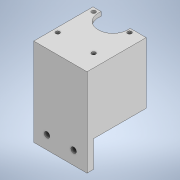
# Autodesk Inventor part: サーボモータ固定用
Saved by Autodesk Inventor 2022 (Build 260153000, 153)
## iProperties
Created: 2022-11-22
Part Number: サーボモータ固定用
Material: 一般
Document SubType Name: Modeling
Designer: tdn82
Density: 1 g/cm^3
Appearance: 既定
Author: tdn82
Autodesk Inventor part; units mm, degrees
ref_plane "YZ Plane" through (0, 0, 0) normal (1, 0, 0) x (0, 1, 0)
ref_plane "XZ Plane" through (0, 0, 0) normal (0, 1, 0) x (-1, 0, 0)
ref_plane "XY Plane" through (0, 0, 0) normal (0, 0, 1) x (1, 0, 0)
sketch "スケッチ1" plane through (0, 0, 0) normal (0, 1, 0) x (-1, 0, 0)
  line L0 (0, 0) -> (-34, 0)
  line L1 (-34, 0) -> (-34, -44.5)
  line L2 (-34, -44.5) -> (0, -44.5)
  line L3 (0, -44.5) -> (0, 0)
  dimension "d0" = 44.5
  dimension "d1" = 34
  constraints: 8 end point, 2 parallel, 1 horizontal, 1 perpendicular
  measures "d0" distance of L2.end L0.start
  measures "d1" distance of L0.start L0.end
extrude "押し出し1" add sketch "スケッチ1" along normal blind 46
sketch "スケッチ2" plane through (34, 0, 0) normal (1, 0, 0) x (0, 0, -1)
  line L0 (3, 43) -> (53, 43)
  line L1 (53, 43) -> (53, 3)
  line L2 (53, 3) -> (3, 3)
  line L3 (3, 3) -> (3, 43)
  line L4 (0, 46) -> (44.5, 46) projected
  line L5 (0, 0) -> (0, 46) projected
  dimension "d4" = 3
  dimension "d5" = 3
  dimension "d6" = 40
  dimension "d7" = 50
  constraints: 8 end point, 2 parallel, 1 horizontal, 1 perpendicular
  measures "d4" distance between parallel lines of L0 L4
  measures "d5" distance between parallel lines of L5 L3
  measures "d6" distance of L2.end L0.start
  measures "d7" distance of L0.start L0.end
extrude "押し出し2" cut sketch "スケッチ2" against normal blind 43.5
sketch "スケッチ3" plane through (0, 0, 0) normal (0, -1, 0) x (1, 0, 0)
  circle A0 centre (17, -42.5) radius 11
  line L0 (34, -44.5) -> (0, -44.5) projected
  line L1 (0, -44.5) -> (0, 0) projected
  point P0 (6.1833, -44.5)
  point P1 (27.8167, -44.5)
  dimension "d10" = 22
  dimension "d11" = 2
  dimension "d12" = 17
  constraints: 1 centre point
  measures "d10" diameter of A0
  measures "d11" distance from line of A0.centre L0
  measures "d12" distance from line of L1 A0.centre
extrude "押し出し3" cut sketch "スケッチ3" against normal blind 3 contours A0 L0 picked at (20.7405, -38.2254)
sketch "スケッチ4" plane through (0, 46, 0) normal (0, 1, 0) x (1, 0, 0)
  circle A0 centre (17, 42.5) radius 11
  line L0 (34, 44.5) -> (0, 44.5) projected
  line L1 (0, 44.5) -> (0, 0) projected
  point P0 (27.8167, 44.5)
  point P1 (6.1833, 44.5)
  point P2 (0, 35.0774)
  dimension "d15" = 22
  dimension "d16" = 2
  dimension "d17" = 17
  constraints: 1 centre point
  measures "d15" diameter of A0
  measures "d16" distance from line of L0 A0.centre
  measures "d17" distance from line of A0.centre L1
extrude "押し出し4" cut sketch "スケッチ4" against normal blind 3
sketch "スケッチ5" plane through (0, 46, 0) normal (0, 1, 0) x (1, 0, 0)
  line L0 (0, 0) -> (34, 0) projected
  line L1 (0, 44.5) -> (0, 0) projected
  line L2 (34, 0) -> (34, 44.5) projected
  point P0 (3.5, 14.5)
  point P1 (3.5, 41.5)
  point P2 (30.5, 41.5)
  point P3 (30.5, 14.5)
  dimension "d20" = 14.5
  dimension "d21" = 3.5
  dimension "d22" = 27
  dimension "d23" = 3.5
  dimension "d48" = 3.5
  dimension "d55" = 14.5
  dimension "d56" = 27
  measures "d20" distance from line of L0 point (3.5, 14.5)
  measures "d21" distance from line of point (3.5, 14.5) L1
  measures "d22" distance of point (3.5, 41.5) point (3.5, 14.5)
  measures "d23" distance from line of L2 point (30.5, 41.5)
  measures "d48" distance from line of point (30.5, 14.5) L2
  measures "d55" distance from line of L0 point (30.5, 14.5)
  measures "d56" distance of point (30.5, 41.5) point (30.5, 14.5)
hole "穴1" at (3.5, 46, -14.5) at (3.5, 46, -41.5) at (30.5, 46, -41.5) at (30.5, 46, -14.5) direction (0, -1, 0) diameter 3 end through all
fillet "フィレット1" radius 2 1 edges at (17, 43, -3)
fillet "フィレット2" radius 2 1 edges at (17, 3, -3)
sketch "スケッチ8" plane through (0, 0, 0) normal (0, 0, 1) x (1, 0, 0)
  line L0 (0, 0) -> (34, 0)
  line L1 (34, 0) -> (34, -20)
  line L2 (34, -20) -> (0, -20)
  line L3 (0, -20) -> (0, 0)
  line L4 (34, 0) -> (34, 46) projected
  dimension "d59" = 20
  constraints: 8 end point, 2 parallel, 1 collinear, 1 horizontal, 1 perpendicular
  measures "d59" distance between parallel lines of L0 L2
extrude "押し出し5" add sketch "スケッチ8" against normal blind 5
sketch "スケッチ9" plane through (0, 0, -5) normal (0, 0, -1) x (-1, 0, 0)
  line L0 (-30, -10) -> (-10, -10)
  line L1 (-34, -20) -> (0, -20) projected
  line L2 (-34, 0) -> (-34, -20) projected
  line L3 (0, -20) -> (0, 0) projected
  point P0 (-17, -20)
  point P1 (-34, -10)
  dimension "d62" = 20
  dimension "d71" = 10
  constraints: 2 coincident, 2 end point, 2 midpoint, 1 horizontal, 1 horizontal alignment
  measures "d62" distance of L0.start L0.end
  measures "d71" distance from line of point (-10, -10) L3
hole "穴3" at (30, -10, -5) at (10, -10, -5) direction (0, 0, 1) diameter 4.134 end through all thread size "M5x0.8" class "6H" standard "ISO Metric profile"
sketch "スケッチ11" plane through (34, 46, 0) normal (1, 0, 0) x (0, 0, -1)
  line L0 (44.5, -43) -> (5, -43) projected
  arc A0 (3, -41) -> (5, -43) centre (5, -41) ccw projected
  line L1 (3, -41) -> (3, -5) projected
  arc A1 (5, -3) -> (3, -5) centre (5, -5) ccw projected
  line L2 (5, -3) -> (44.5, -3) projected
  line L3 (44.5, -3) -> (44.5, 0) projected
  line L4 (0, 0) -> (44.5, 0) projected
  line L5 (0, -66) -> (0, 0) projected
  line L6 (0, -66) -> (5, -66) projected
  line L7 (5, -46) -> (5, -66) projected
  line L8 (5, -46) -> (44.5, -46) projected
  line L9 (44.5, -46) -> (44.5, -43) projected
  point P0 (0, -46)
extrude "押し出し6" add sketch "スケッチ11" along normal blind 6
sketch "スケッチ12" plane through (40, 46, 0) normal (1, 0, 0) x (0, 0, -1)
  line L0 (5, -46) -> (44.5, -46) projected
  line L1 (44.5, -46) -> (0, -46)
  line L2 (0, -46) -> (0, 0)
  line L3 (0, 0) -> (44.5, 0)
  line L4 (44.5, 0) -> (44.5, -46)
  constraints: 8 end point, 2 parallel, 1 horizontal, 1 perpendicular
extrude "押し出し7" add sketch "スケッチ12" against normal blind 4
